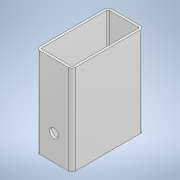
# Autodesk Inventor part: tubo1-40x40x640
Saved by Autodesk Inventor 2021.2 (Build 252289000, 289)
## iProperties
Created: 2026-06-02
Part Number: tubo1-40x40x640
Material: Aluminum
Document SubType Name: Modeling
Designer: nelso
Density: 2.7 g/cm^3
Appearance: Satin
Author: nelso
Autodesk Inventor part; units mm, degrees
ref_plane "YZ Plane" through (0, 0, 0) normal (1, 0, 0) x (0, 1, 0)
ref_plane "XZ Plane" through (0, 0, 0) normal (0, 1, 0) x (-1, 0, 0)
ref_plane "XY Plane" through (0, 0, 0) normal (0, 0, 1) x (1, 0, 0)
sketch "Sketch1" plane through (0, 0, 0) normal (0, 1, 0) x (-1, 0, 0)
  line L0 (-20, 40) -> (20, 40)
  line L1 (20, 40) -> (20, -40)
  line L2 (20, -40) -> (-20, -40)
  line L3 (-20, -40) -> (-20, 40)
  line L4 (-20, 40) -> (20, -40) construction
  line L5 (20, 40) -> (-20, -40) construction
  line L6 (-17.5, 37.5) -> (17.5, 37.5)
  line L7 (17.5, 37.5) -> (17.5, -37.5)
  line L8 (17.5, -37.5) -> (-17.5, -37.5)
  line L9 (-17.5, -37.5) -> (-17.5, 37.5)
  line L10 (-17.5, 37.5) -> (17.5, -37.5) construction
  line L11 (17.5, 37.5) -> (-17.5, -37.5) construction
  point P0 (0, 0)
  dimension "d0" = 40
  dimension "d1" = 80
  dimension "d30" = 2.5
  dimension "d31" = 2.5
  constraints: 24 end point, 4 midpoint, 4 parallel, 2 horizontal, 2 perpendicular
  measures "d0" distance of L1.end L2.end
  measures "d1" distance of L0.end L1.end
  measures "d30" distance between parallel lines of L8 L2
  measures "d31" distance between parallel lines of L3 L9
extrude "Extrusion1" add sketch "Sketch1" along normal mid plane 100
fillet "Fillet1" radius 3.75 4 edges at (20, 0, -40) (20, 0, 40) (-20, 0, -40) (-20, 0, 40)
fillet "Fillet1" radius 1.25 4 edges at (17.5, 0, -37.5) (-17.5, 0, -37.5) (-17.5, 0, 37.5) (17.5, 0, 37.5)
sketch "Sketch2" plane through (16.25, 50, -40) normal (0, 0, -1) x (-1, 0, 0)
  line L0 (32.5, -100) -> (0, -100) projected
  line L1 (16.25, -100) -> (16.25, -71.5)
  circle A0 centre (16.25, -71.5) radius 4.95
  circle A1 centre (16.25, -71.5) radius 10
  point P0 (16.25, -50)
  dimension "d10" = 28.5
  dimension "d11" = 9.9
  dimension "d12" = 20
  constraints: 2 centre point, 2 coincident, 2 end point, 1 midpoint, 1 vertical
  measures "d10" distance of L1.start L1.end
  measures "d11" diameter of A0
  measures "d12" diameter of A1
extrude "Extrusion2" cut sketch "Sketch2" against normal through all contours A0
sketch "Sketch3" plane through (16.25, 50, -40) normal (0, 0, -1) x (-1, 0, 0)
  circle A0 centre (16.25, -71.5) radius 4.95 projected
  circle A1 centre (16.25, -71.5) radius 10
  point P0 (16.25, -50)
  dimension "d15" = 20
  constraints: 1 centre point, 1 coincident
  measures "d15" diameter of A1
extrude "Extrusion3" cut sketch "Sketch3" against normal blind 10
equation "\"d31\" = d30"
body "Solid1"
